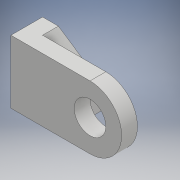
# Autodesk Inventor part: 27
Saved by Autodesk Inventor 2017 (Build 210142000, 142)
## iProperties
Part Number: 27
Material: 一般
Document SubType Name: Modeling
Designer: Brian
Density: 1 g/cm^3
Appearance: 預設
Author: Brian
Autodesk Inventor part; units mm, degrees
ref_plane "YZ Plane" through (0, 0, 0) normal (1, 0, 0) x (0, 1, 0)
ref_plane "XZ Plane" through (0, 0, 0) normal (0, 1, 0) x (-1, 0, 0)
ref_plane "XY Plane" through (0, 0, 0) normal (0, 0, 1) x (1, 0, 0)
sketch "草圖1" plane through (0, 0, 0) normal (0, 1, 0) x (-1, 0, 0)
  line L0 (0, 0) -> (-70, 0)
  line L1 (-70, 0) -> (-70, -40)
  line L2 (-70, -40) -> (0, -40)
  line L3 (0, -40) -> (0, 0)
  dimension "d0" = 40
  dimension "d1" = 70
  constraints: 8 end point, 2 parallel, 1 horizontal, 1 perpendicular
  measures "d0" distance of L2.end L0.start
  measures "d1" distance of L1.end L2.end
extrude "擠出1" add sketch "草圖1" along normal blind 10
sketch "草圖2" plane through (0, 10, 0) normal (0, 1, 0) x (1, 0, 0)
  line L0 (0, 0) -> (70, 0) projected
  line L1 (70, 40) -> (0, 40) projected
  line L2 (0, 0) -> (30, 0)
  line L3 (30, 0) -> (30, 40)
  line L4 (30, 40) -> (0, 40)
  line L5 (0, 40) -> (0, 0)
  dimension "d4" = 30
  constraints: 8 end point, 2 parallel, 1 horizontal, 1 perpendicular, 1 point on line
  measures "d4" distance between parallel lines of L5 L3
extrude "擠出2" add sketch "草圖2" along normal blind 20
sketch "草圖3" plane through (0, 30, 0) normal (0, 1, 0) x (1, 0, 0)
  line L0 (30, 30) -> (10, 0)
  line L1 (0, 0) -> (70, 0) projected
  line L2 (30, 0) -> (30, 30)
  line L3 (30, 0) -> (30, 40) projected
  line L4 (30, 0) -> (10, 0)
  dimension "d7" = 20
  dimension "d8" = 30
  constraints: 6 end point, 3 collinear, 1 point on line
  measures "d7" distance of L2.start L0.end
  measures "d8" vertical distance of L0.start L0.end
extrude "擠出3" cut sketch "草圖3" against normal blind 20
sketch "草圖4" plane through (0, 0, -40) normal (-1, 0, 0) x (0, 0, 1)
  line L0 (-20, 30) -> (40, 30)
  line L1 (10, 30) -> (40, 20)
  line L2 (40, 0) -> (40, 30) projected
  dimension "d11" = 10
  dimension "d12" = 30
  constraints: 4 end point, 1 midpoint, 1 point on line
  measures "d11" vertical distance of L1.start L1.end
  measures "d12" horizontal distance of L1.start L1.end
extrude "擠出4" cut sketch "草圖4" against normal through all
fillet "圓角1" radius 20 2 edges at (70, 5, 0) (70, 5, -40)
hole "孔1" at (50, 10, -20) direction (0, -1, 0) diameter 20 depth 10 tip angle 118
